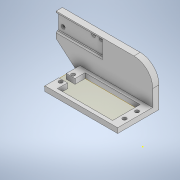
# Autodesk Inventor part: servov2
Saved by Autodesk Inventor 2021 (Build 250183000, 183)
## iProperties
Created: 2022-04-18
Part Number: servov2
Material: Genérico
Document SubType Name: Modeling
Designer: orgyn
Density: 1 g/cm^3
Appearance: Valor por defecto
Author: orgyn
Autodesk Inventor part; units mm, degrees
ref_plane "YZ Plane" through (0, 0, 0) normal (1, 0, 0) x (0, 1, 0)
ref_plane "XZ Plane" through (0, 0, 0) normal (0, 1, 0) x (-1, 0, 0)
ref_plane "XY Plane" through (0, 0, 0) normal (0, 0, 1) x (1, 0, 0)
ref_plane "Plano de trabajo1" through (0, 27, 0) normal (0, 1, 0) x (1, 0, 0)
sketch "Boceto2" plane through (0, 27, 0) normal (0, 1, 0) x (1, 0, 0)
  line L0 (0, 10) -> (0, 15)
  line L1 (0, 15) -> (11.8906, 15)
  line L2 (0, 10) -> (0, 5)
  line L3 (0, 5) -> (15.0689, 5)
  line L4 (0, 5) -> (7, 5)
  line L5 (7, 5) -> (7, 15)
  line L6 (6.4875, 15) -> (4.4875, 15)
  circle A0 centre (4.4875, 15) radius 1.5
  circle A1 centre (4.4875, 5) radius 1.5
  line L7 (-42, 6) -> (-42, 0) projected
  line L8 (0, 0) -> (-42, 0)
  line L9 (-42, 0) -> (0, 0) projected
  line L10 (-21, 0) -> (-21, 36.5425)
  circle A2 centre (-46.4875, 15) radius 1.5
  circle A3 centre (-46.4875, 5) radius 1.5
  line L11 (0, 0) -> (1, 0)
  line L12 (1, 0) -> (8, 0)
  line L13 (8, 0) -> (8, 20)
  line L14 (8, 20) -> (1, 20)
  line L15 (1, 20) -> (1, 0)
  line L16 (-42, 10) -> (-42, 15)
  line L17 (-42, 15) -> (-53.8906, 15)
  line L18 (-42, 10) -> (-42, 5)
  line L19 (-42, 5) -> (-49, 5)
  line L20 (-49, 5) -> (-49, 15)
  line L21 (-48.4875, 15) -> (-46.4875, 15)
  circle A4 centre (-46.4875, 15) radius 1.5
  circle A5 centre (-46.4875, 5) radius 1.5
  line L22 (-42, 0) -> (-43, 0)
  line L23 (-43, 0) -> (-50, 0)
  line L24 (-50, 0) -> (-50, 20)
  line L25 (-50, 20) -> (-43, 20)
  line L26 (-43, 20) -> (-43, 0)
  line L27 (-43, 20) -> (-43, 21)
  line L28 (-43, 21) -> (1, 21)
  line L29 (1, 21) -> (1, 20)
  line L30 (-43, 0) -> (-43, -1)
  line L31 (-43, -1) -> (1, -1)
  line L32 (1, -1) -> (1, 0)
  line L33 (-50, 20) -> (-50, 24)
  line L34 (-50, 24) -> (8, 24)
  line L35 (-50, 0) -> (-50, -4)
  line L36 (-50, -4) -> (8, -4)
  line L37 (8, -4) -> (8, 0)
  line L38 (8, 24) -> (8, 19.2948)
  line L39 (-42, 10) -> (-42, 7)
  line L40 (-42, 7) -> (-58.0956, 7)
  line L41 (-51, 14) -> (-51, 6) projected
  line L42 (-42, 10) -> (-42, 13)
  line L43 (-42, 13) -> (-56.402, 13)
  point P0 (0, 20)
  point P1 (-42, 20)
  point P2 (-50, 13)
  point P3 (-43, 13)
  point P4 (-43, 7)
  point P5 (-50, 7)
  dimension "d8" = 5
  dimension "d9" = 5
  dimension "d10" = 7
  dimension "d11" = 2
  dimension "d12" = 3
  dimension "d13" = 3
  dimension "d14" = 1
  dimension "d15" = 7
  dimension "d16" = 1
  dimension "d17" = 1
  dimension "d18" = 4
  dimension "d19" = 4
  dimension "d22" = 3
  dimension "d23" = 3
  constraints: 82 end point, 17 symmetric about line, 16 point on line, 12 perpendicular, 6 centre point, 4 vertical, 2 coincident, 1 horizontal, 1 midpoint, 1 parallel, 4 other
  measures "d8" distance of L0.start L0.end
  measures "d9" distance of L0.start L2.end
  measures "d10" distance of L2.end L4.end
  measures "d11" distance of L6.start L6.end
  measures "d12" diameter of A0
  measures "d13" diameter of A1
  measures "d14" distance of L8.start L11.end
  measures "d15" distance of L11.end L12.end
  measures "d16" distance of L26.start L27.end
  measures "d17" distance of L22.end L30.end
  measures "d18" distance of L24.end L33.end
  measures "d19" distance of L23.end L35.end
  measures "d22" distance of L16.start L39.end
  measures "d23" distance of L16.start L42.end
extrude "Extrusión2" add sketch "Boceto2" along normal blind 4 contours L15 L14 L13 L1 A0 | L1 A0 L5 L3 A1 L15 | L3 A1 L13 L12 L15 | L29 L28 L10 L34 L38 L14 | L12 L37 L36 L35 L23 L30 L31 L32 | L28 L27 L25 L33 L34 L10 | L5 L1 L13 L3 | L23 L24 L40 L20 L19 A3 L26 | L26 L17 A2 L24 L25 | L19 A3 L20 L40 L26 | L26 L43 L20 L17 A2 | L17 L20 L43 L24
sketch "Boceto3" plane through (8, 27, -24) normal (0, 0, -1) x (-1, 0, 0)
  point P0 (8, -27)
sketch "Boceto4" plane through (8, 27, -24) normal (0, 0, -1) x (-1, 0, 0)
  line L0 (0, 4) -> (58, 4) projected
  line L1 (58, 4) -> (58, 18.1)
  line L2 (58, 18.1) -> (0, 18.1)
  line L3 (0, 18.1) -> (0, 4)
  line L4 (58, 18.1) -> (58, 22.1)
  line L5 (58, 18.1) -> (58, 32.1)
  line L6 (58, 32.1) -> (0, 32.1)
  line L7 (0, 32.1) -> (0, 18.1)
  line L8 (58, 18.1) -> (58, 28.6)
  line L9 (58, 28.6) -> (36.9156, 28.6)
  line L10 (8, -6.3468) -> (8, 18.1)
  line L11 (8, 18.1) -> (18.1, 18.1)
  line L12 (18.1, 18.1) -> (41.1, 18.1)
  line L13 (41.1, 18.1) -> (51.1, 18.1)
  line L14 (51.1, 18.1) -> (51.1, 26.6579)
  line L15 (51.1, 26.6579) -> (51.1, 31.1823)
  line L16 (51.1, 18.1) -> (51.1, 18)
  line L17 (51.1, 18.1) -> (51.2, 18.1)
  line L18 (51.2, 18.1) -> (51.2, 31.1)
  line L19 (51.2, 31.1) -> (41.1, 31.1)
  line L20 (41.1, 31.1) -> (41.1, 18.1)
  line L21 (51.2, 28.6) -> (49.2, 28.6)
  line L22 (41.1, 28.6) -> (43.1, 28.6)
  line L23 (43.1, 28.6) -> (43.15, 28.6)
  circle A0 centre (43.15, 28.6) radius 1.5
  line L24 (43.15, 28.6) -> (49.15, 28.6)
  circle A1 centre (49.15, 28.6) radius 1.5
  point P0 (8, -27)
  point P1 (8, 4)
  dimension "d24" = 14.1
  dimension "d25" = 4
  dimension "d26" = 14
  dimension "d27" = 10.5
  dimension "d28" = 10.1
  dimension "d29" = 23
  dimension "d30" = 10
  dimension "d31" = 0.1
  dimension "d32" = 0.1
  dimension "d33" = 13
  dimension "d34" = 10.1
  dimension "d35" = 2
  dimension "d36" = 2
  dimension "d38" = 0.05
  dimension "d39" = 3
  dimension "d40" = 6
  dimension "d41" = 3
  constraints: 48 end point, 16 point on line, 9 perpendicular, 3 vertical, 2 centre point, 2 coincident
  measures "d24" distance of L0.end L1.end
  measures "d25" distance of L1.end L4.end
  measures "d26" distance of L1.end L5.end
  measures "d27" distance of L1.end L8.end
  measures "d28" distance of L10.end L11.end
  measures "d29" distance of L11.end L12.end
  measures "d30" distance of L12.end L13.end
  measures "d31" distance of L13.end L16.end
  measures "d32" distance of L13.end L17.end
  measures "d33" distance of L17.end L18.end
  measures "d34" distance of L18.end L19.end
  measures "d35" distance of L21.start L21.end
  measures "d36" distance of L22.start L22.end
  measures "d38" distance of L22.end L23.end
  measures "d39" diameter of A0
  measures "d40" distance of L24.start L24.end
  measures "d41" diameter of A1
extrude "Extrusión3" add sketch "Boceto4" along normal blind 5 contours L3 L2 L10 L0 | L10 L2 L1 L0 | L7 L6 L5 L9 L18 L19 L20 L2 | L2 L18 L9 L5 L4
sketch "Boceto5" plane through (8, 27, -29) normal (0, 0, -1) x (-1, 0, 0)
  line L0 (51.2, 18.1) -> (41.1, 18.1) projected
  line L1 (51.2, 18.1) -> (51.2, 28.6)
  line L2 (51.2, 31.1) -> (51.2, 18.1) projected
  line L3 (51.2, 28.6) -> (49.15, 28.6)
  circle A0 centre (49.15, 28.6) radius 1.5
  line L4 (49.15, 28.6) -> (43.15, 28.6)
  circle A1 centre (43.15, 28.6) radius 1.5
  line L5 (41.1, 18.1) -> (51.2, 18.1)
  line L6 (51.2, 18.1) -> (51.2, 31.1)
  line L7 (51.2, 31.1) -> (41.1, 31.1)
  line L8 (41.1, 31.1) -> (41.1, 18.1)
  point P0 (8, -27)
  dimension "d44" = 10.5
  dimension "d45" = 2.05
  dimension "d46" = 3
  dimension "d47" = 6
  dimension "d48" = 3
  constraints: 14 end point, 2 centre point, 2 coincident, 2 horizontal, 2 parallel, 2 perpendicular, 1 point on line
  measures "d44" distance of L0.start L1.end
  measures "d45" distance of L1.end L3.end
  measures "d46" diameter of A0
  measures "d47" distance of L4.start L4.end
  measures "d48" diameter of A1
extrude "Extrusión4" add sketch "Boceto5" against normal blind 3
sketch "Boceto6" plane through (-50, 31, -24) normal (0, -1, 0) x (1, 0, 0)
  line L0 (58, -5) -> (0, -5) projected
  line L1 (0, 0) -> (58, 0)
  line L2 (58, 0) -> (58, -5)
  line L3 (58, -5) -> (0, -5)
  line L4 (0, -5) -> (0, 0)
  point P0 (50, 24)
  constraints: 8 end point, 2 parallel, 1 horizontal, 1 perpendicular
extrude "Extrusión5" add sketch "Boceto6" along normal blind 4
sketch "Boceto7" plane through (8, 27, -24) normal (0, 0, 1) x (1, 0, 0)
  line L0 (-51.2, 31.1) -> (-72.2407, 31.1)
  line L1 (-51.2, 31.1) -> (-51.2, 18.1) projected
  line L2 (-51.2, 18.1) -> (-72.8631, 18.1)
  line L3 (-72.8631, 18.1) -> (-72.2407, 31.1)
  point P0 (-8, -27)
  constraints: 6 end point, 2 horizontal
extrude "Extrusión6" cut sketch "Boceto7" against normal blind 2
sketch "Boceto8" plane through (-50, 27, -13) normal (-1, 0, 0) x (0, 0, 1)
  line L0 (-11, 31.1) -> (-11, 32.1) projected
  line L1 (-11, 32.1) -> (-11, 31.1)
  line L2 (-11, 31.1) -> (-13, 31.1)
  line L3 (-13, 18.1) -> (-13, 31.1) projected
  line L4 (-13, 31.1) -> (-13, 18.1)
  line L5 (-11, 18.1) -> (-13, 18.1) projected
  line L6 (-13, 18.1) -> (-11, 18.1)
  line L7 (-11, 18.1) -> (-11, 0.1456)
  line L8 (-11, 0.1456) -> (-11, 0)
  line L9 (0, 0) -> (-16, 0) projected
  line L10 (-16, 32.1) -> (-16, 0) projected
  line L11 (-11, 0) -> (-16, 0)
  line L12 (-16, 0) -> (-16, 32.1)
  line L13 (-11, 32.1) -> (-16, 32.1) projected
  line L14 (-16, 32.1) -> (-11, 32.1)
  point P0 (13, -27)
  point P1 (-13, 31.1)
  constraints: 18 end point, 4 collinear, 3 point on line, 1 horizontal, 1 perpendicular, 1 vertical
extrude "Extrusión7" add sketch "Boceto8" along normal blind 19.1
sketch "Boceto10" plane through (8, 27, -24) normal (0, 0, 1) x (1, 0, 0)
  line L0 (-77.1, 18.1) -> (-73.389, 18.1)
  line L1 (-77.1, 18.1) -> (-41.1, 18.1) projected
  line L2 (-73.389, 18.1) -> (-73.389, 22.1)
  circle A0 centre (-73.389, 22.1) radius 1.5
  point P0 (-8, -27)
  dimension "d62" = 3.711
  dimension "d63" = 4
  dimension "d64" = 3
  constraints: 4 end point, 1 centre point, 1 coincident, 1 perpendicular, 1 point on line
  measures "d62" distance of L0.start L0.end
  measures "d63" distance of L0.end L2.end
  measures "d64" diameter of A0
extrude "Extrusión9" cut sketch "Boceto10" against normal blind 19.1
sketch "Boceto11" plane through (8, 27, -24) normal (0, 0, 1) x (1, 0, 0)
  line L0 (-58, 0) -> (-77.1, 0) projected
  line L1 (-58, 0) -> (-77.1, 13.1321)
  line L2 (-77.1, 0) -> (-77.1, 18.1) projected
  line L3 (-58, 0) -> (-77.1, 0)
  line L4 (-77.1, 0) -> (-77.1, 13.1321)
  line L5 (-61.7227, 0) -> (-77.1, 13.1321)
  line L6 (-61.7227, 0) -> (-77.1, 0)
  point P0 (-8, -27)
  constraints: 10 end point, 2 horizontal, 2 point on line, 1 perpendicular
extrude "Extrusión10" cut sketch "Boceto11" against normal blind 19.1 contours L0 L2 L5
fillet "Empalme1" radius 15 1 edges at (8, 59.1, -26.5)
chamfer "Chaflán1" distance 1 angle 45 2 edges at (-51.1, 45.1, -24) (-33.1, 51.6, -24)
